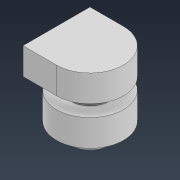
# Autodesk Inventor part: Table Hinge
Saved by Autodesk Inventor 2021 (Build 250183000, 183)
## iProperties
Created: 2021-01-30
Part Number: Table Hinge
Material: Generic
Document SubType Name: Modeling
Designer: PaisW
Density: 1 g/cm^3
Appearance: Default
Author: PaisW
Autodesk Inventor part; units mm, degrees
ref_plane "YZ Plane" through (0, 0, 0) normal (1, 0, 0) x (0, 1, 0)
ref_plane "XZ Plane" through (0, 0, 0) normal (0, 1, 0) x (-1, 0, 0)
ref_plane "XY Plane" through (0, 0, 0) normal (0, 0, 1) x (1, 0, 0)
sketch "Sketch1" plane through (0, 0, 0) normal (0, 1, 0) x (-1, 0, 0)
  line L0 (13.075, -26.15) -> (-13.075, -26.15)
  line L1 (-13.075, -26.15) -> (-13.075, 26.15)
  line L2 (-13.075, 26.15) -> (13.075, 26.15)
  line L3 (13.075, 26.15) -> (13.075, -26.15)
  arc A0 (-13.075, 26.15) -> (-13.075, -26.15) centre (-13.075, 0) ccw
  circle A1 centre (-13.075, 0) radius 26.15
  point P0 (0, 0)
  point P1 (0, -26.15)
  dimension "d0" = 26.15
  constraints: 8 end point, 2 midpoint, 2 parallel, 2 point on circle, 2 vertical alignment, 1 centre point, 1 coincident, 1 horizontal, 1 horizontal alignment, 1 perpendicular, 1 tangent, 1 vertical, 2 other
  measures "d0" radius of A0
extrude "Extrusion1" add sketch "Sketch1" along normal blind 20.8
sketch "Sketch2" plane through (0, 20.8, 0) normal (0, 1, 0) x (1, 0, 0)
  circle A0 centre (13.075, 0) radius 15
  arc A1 (13.075, -26.15) -> (13.075, 26.15) centre (13.075, 0) ccw projected
  point P0 (0, 0)
  dimension "d3" = 30
  constraints: 1 centre point, 1 concentric
  measures "d3" diameter of A0
extrude "Extrusion2" add sketch "Sketch2" along normal blind 9.3
sketch "Sketch3" plane through (0, 0, 0) normal (0, -1, 0) x (1, 0, 0)
  circle A0 centre (13.075, 0) radius 15
  arc A1 (13.075, -26.15) -> (13.075, 26.15) centre (13.075, 0) ccw projected
  point P0 (0, 0)
  dimension "d6" = 30
  constraints: 1 centre point, 1 concentric
  measures "d6" diameter of A0
extrude "Extrusion3" add sketch "Sketch3" along normal blind 9
sketch "Sketch4" plane through (13.075, 30.1, 0) normal (0, 1, 0) x (1, 0, 0)
  line L0 (-26.15, 26.15) -> (-26.15, -26.15) projected
  line L1 (-26.15, -26.15) -> (-26.15, 26.15)
  line L2 (0, 26.15) -> (-26.15, 26.15) projected
  line L3 (-26.15, 26.15) -> (0, 26.15)
  arc A0 (0, -26.15) -> (0, 26.15) centre (0, 0) ccw projected
  arc A1 (0, -26.15) -> (0, 26.15) centre (0, 0) ccw
  line L4 (-26.15, -26.15) -> (0, -26.15) projected
  line L5 (0, -26.15) -> (-26.15, -26.15)
  point P0 (-13.075, 0)
  constraints: 6 end point, 2 collinear, 2 point on circle, 1 centre point, 1 concentric, 1 vertical
extrude "Extrusion4" add sketch "Sketch4" along normal blind 20.8
fillet "Fillet1" radius 26.15 2 edges at (-13.075, 10.4, -26.15) (-13.075, 10.4, 26.15)
body "Solid1"
